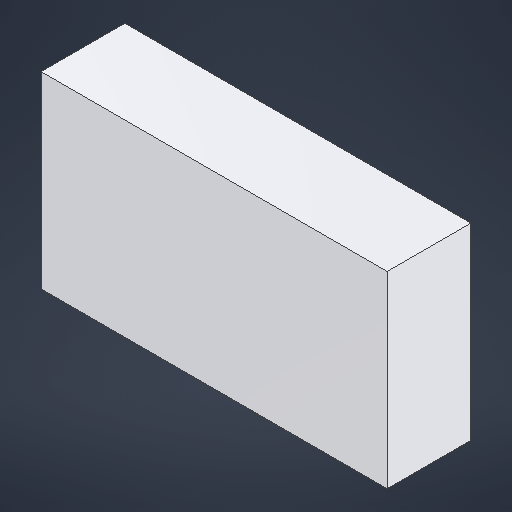
# Autodesk Inventor part: battery_case
Saved by Autodesk Inventor 2026.2 (Build 302298010, 298A)
## iProperties
Created: 2026-07-05
Part Number: battery_case
Material: Generic
Document SubType Name: Modeling
Designer: vicke
Density: 1 g/cm^3
Appearance: Default
Author: vicke
Autodesk Inventor part; units mm, degrees
ref_plane "YZ Plane" through (0, 0, 0) normal (1, 0, 0) x (0, 1, 0)
ref_plane "XZ Plane" through (0, 0, 0) normal (0, 1, 0) x (-1, 0, 0)
ref_plane "XY Plane" through (0, 0, 0) normal (0, 0, 1) x (1, 0, 0)
sketch "Sketch1" plane through (0, 0, 0) normal (0, 0, 1) x (1, 0, 0)
  line L0 (0, 0) -> (75.6, 0)
  line L1 (75.6, 0) -> (75.6, 41.1)
  line L2 (75.6, 41.1) -> (0, 41.1)
  line L3 (0, 41.1) -> (0, 0)
  dimension "d0" = 75.6
  dimension "d1" = 41.1
  constraints: 8 end point, 2 parallel, 1 horizontal, 1 perpendicular
  measures "d0" distance between parallel lines of L1 L3
  measures "d1" distance between parallel lines of L0 L2
extrude "Extrusion1" add sketch "Sketch1" along normal blind 18.3
body "Solid1"
